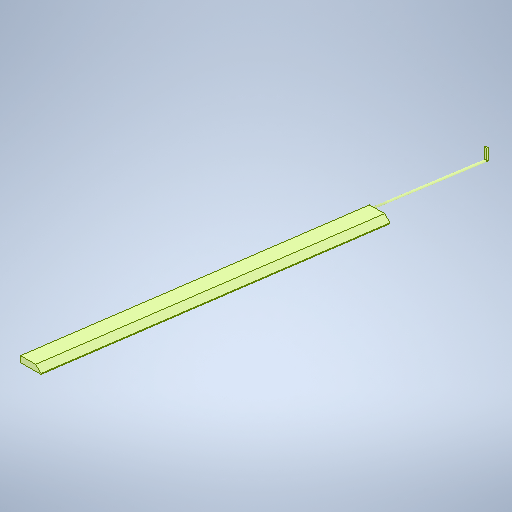
# Autodesk Inventor part: ALA
Saved by Autodesk Inventor 2025.3 (Build 293356030, 356C)
## iProperties
Created: 2025-07-04
Part Number: ALA
Material: Generic
Document SubType Name: Modeling
Designer: steve
Density: 1 g/cm^3
Appearance: Default(2)
Author: steve
Autodesk Inventor part; units mm, degrees
sketch "Sketch1" plane through (0, 0, 0) normal (0, 0, 1) x (1, 0, 0)
  line L0 (0, 0) -> (240, 0)
  line L1 (240, 1.3) -> (240, -1.3)
  line L2 (0, 0) -> (0, 11.6325) construction
  line L3 (0, 11.6325) -> (63.9666, 39.9868) construction
  line L4 (63.9666, 39.9868) -> (240, 1.3) construction
  spline S0 degree 3 poles (0, 0) (0, 11.6325) (63.9666, 39.9868) (240, 1.3) knots 1 1 1 1 2 2 2 2
  line L5 (0, 0) -> (-1.5698, -20.1343) construction
  line L6 (-1.5698, -20.1343) -> (240, -1.3) construction
  spline S1 degree 2 poles (0, 0) (-1.5698, -20.1343) (240, -1.3) knots 1 1 1 2 2 2
  line L7 (10, 0) -> (10, 9.15)
  line L8 (10, 0) -> (10, -6.78)
  line L9 (90, 0) -> (90, 21.9)
  line L10 (90, 0) -> (90, -10.42)
  dimension "d0" = 240
  dimension "d1" = 2.6
  dimension "d2" = 10
  dimension "d3" = 90
  dimension "d4" = 9.15
  dimension "d5" = 6.78
  dimension "d6" = 21.9
  dimension "d7" = 10.42
  constraints: 12 end point, 5 vertical, 2 point on line, 1 horizontal, 1 midpoint, 6 other
  measures "d0" distance of L0.end L0.start
  measures "d1" distance of L1.start L1.end
  measures "d2" distance of L0.start L7.start
  measures "d3" distance of L0.start L9.start
  measures "d4" distance of L7.start L7.end
  measures "d5" distance of L8.end L7.start
  measures "d6" distance of L9.end L9.start
  measures "d7" distance of L10.end L9.start
sketch "Sketch2" plane through (0, 0, 0) normal (0, 1, 0) x (-1, 0, 0)
  line L0 (0, 0) -> (0, 555)
  line L1 (0, 555) -> (-160, 555)
  line L2 (-160, 555) -> (-240, 0)
  dimension "d8" = 555
  dimension "d9" = 160
  constraints: 6 end point, 1 horizontal, 1 vertical
  measures "d8" distance of L0.start L0.end
  measures "d9" distance of L0.end L1.end
ref_plane "Work Plane2" through (0, 0, 555) normal (0, 0, 1) x (1, 0, 0)
ref_plane "Work Plane4" through (120.002, 10.5253, 0) normal (0, 0, -1) x (-1, 0, 0)
ref_plane "Work Plane5" through (88, -10.0773, 0) normal (0, 0, -1) x (-1, 0, 0)
ref_plane "Work Plane3" through (240, -1.3, 0) normal (0, 0, -1) x (-1, 0, 0)
ref_plane "Work Plane6" through (192.6847, -3.2567, 134) normal (0, 0, 1) x (1, 0, 0)
sketch "Sketch8" plane through (192.6847, -3.2567, 134) normal (0, 0, 1) x (1, 0, 0)
  circle A0 centre (3, 4.8257) radius 1.25
  line L0 (0, 9.6514) -> (0, 0) projected
  point P0 (-192.6847, 3.2567)
  point P1 (0, 4.8257)
  dimension "d36" = 2.5
  dimension "d37" = 3
  dimension "d38" = 9.6514
  constraints: 1 centre point, 1 horizontal alignment, 1 midpoint
  measures "d36" diameter of A0
  measures "d37" distance from line of A0.centre L0
  measures "d38" distance of L0.start L0.end
sketch "Sketch9" plane through (240, -1.3, 0) normal (0, 0, -1) x (-1, 0, 0)
  circle A0 centre (25, 1.3) radius 1.5
  line L0 (0, 0) -> (0, 2.6) projected
  point P0 (240, 1.3)
  point P1 (0, 1.3)
  point P2 (0, 1.3)
  dimension "d39" = 25
  dimension "d40" = 3
  constraints: 2 midpoint, 1 centre point, 1 horizontal alignment
  measures "d39" distance of point (0, 1.3) A0.centre
  measures "d40" diameter of A0
loft "Loft2" add profiles "Sketch8", "Sketch9"
sketch "Sketch10" plane through (0, 0, 0) normal (0, 1, 0) x (-1, 0, 0)
  line L0 (-192.6847, 134) -> (-220.6847, 134) projected
  line L1 (-134.1622, 540) -> (-192.6847, 134) projected
  line L2 (-162.1622, 540) -> (-134.1622, 540) projected
  line L3 (-162.1622, 540) -> (-220.6847, 134)
  line L4 (-134.5946, 537) -> (-162.5946, 537)
  line L5 (-135.6049, 537) -> (-193.695, 134)
  point P0 (0, 0)
  point P1 (-220.2523, 137)
  point P2 (-193.2626, 137)
  dimension "d58" = 3
  dimension "d59" = 1
  constraints: 6 end point, 6 point on line, 2 parallel
  measures "d58" distance between parallel lines of L2 L4
  measures "d59" distance between parallel lines of L1 L5
extrude "Extrusion4" add sketch "Sketch10" along normal blind 5 and the other way blind 3 contours L0 L3 L4 L5
chamfer "Chamfer1" distance 7 angle 45 1 edges at (191.6396, 5, 335.5)
sketch "Sketch13" plane through (0, 0, 0) normal (0, 1, 0) x (-1, 0, 0)
  line L0 (-196.9347, 134) -> (-194.4347, 134) projected
  line L1 (-213.5, 0) -> (-216.5, 0) projected
  line L2 (-213.5, 0) -> (-216.5, 0) projected
  line L3 (-213.5, 0) -> (-213.2396, 2.1617)
  line L4 (-213.2396, 2.1617) -> (-216.2396, 2.1617)
  line L5 (-216.2396, 2.1617) -> (-216.5, 0)
  point P0 (0, 0)
  constraints: 6 end point, 2 parallel
extrude "Extrusion5" add sketch "Sketch13" along normal blind 15
sketch "Sketch14" plane through (0, 0, 0) normal (0, 1, 0) x (-1, 0, 0)
  line L0 (-192.6847, 134) -> (-134.1622, 540) projected
  line L1 (-192.6847, 134) -> (-213.5, -10.4063)
  line L2 (-210.5, 0) -> (-216.5, 0) projected
  line L3 (-195.7157, 134) -> (-137.1932, 540) projected
  point P0 (0, 0)
  point P1 (-213.5, 0)
  point P2 (-215.031, 0)
  dimension "d56" = 3
  constraints: 2 end point, 1 collinear, 1 midpoint, 1 vertical alignment
  measures "d56" distance between parallel lines of L0 L3
body "Solid1"
